lego-tray-middle-short (Autodesk Fusion 360 design; units mm, degrees)
Autodesk Fusion 360 part; units mm, degrees
sketch "Sketch1" plane through (0, 0, 0) normal (0, 1, 0) x (1, 0, 0)
  line L0 (0, 0) -> (-127, 0)
  line L1 (-127, 0) -> (-127, 103.0224)
  line L2 (-127, 103.0224) -> (0, 103.0224)
  line L3 (0, 103.0224) -> (0, 0)
  dimension "d1" = 103.0224
  dimension "d2" = 127
  constraint horizontal L0
  constraint vertical L1
  constraint horizontal L2
  constraint vertical L3
  constraint coincident L0.start L3.end
  measures "d1" distance of L0.start L2.end
  measures "d2" distance of L0.start L0.end
extrude "Extrude1" add sketch "Sketch1" along normal blind 38.1 makes body 1
draft "Draft1" [suppressed]
fillet "Fillet1" [suppressed]
fillet "Fillet2" radius 6.35 4 edges at (-127, 19.05, -103.0224) (-127, 19.05, 0) (0, 19.05, 0) (0, 19.05, -103.0224) on bodies 1
fillet "Fillet3" radius 3.175 8 edges at (-125.1401, 0, -1.8599) (-127, 0, -51.5112) (-125.1401, 0, -101.1625) (-63.5, 0, -103.0224) (-1.8599, 0, -101.1625) (0, 0, -51.5112) (-1.8599, 0, -1.8599) (-63.5, 0, 0) on bodies 1
shell "Shell1" thickness 1.524 removed faces 1 at (-44.45, 38.1, -34.3408) on bodies 1
sketch "Sketch2" plane through (0, 38.1, 0) normal (0, 1, 0) x (-1, 0, 0)
  arc A0 (6.35, -1.524) -> (1.524, -6.35) centre (6.35, -6.35) ccw
  line L0 (6.35, -1.524) -> (120.65, -1.524)
  arc A1 (125.476, -6.35) -> (120.65, -1.524) centre (120.65, -6.35) ccw
  line L1 (125.476, -6.35) -> (125.476, -96.6724)
  arc A2 (120.65, -101.4984) -> (125.476, -96.6724) centre (120.65, -96.6724) ccw
  line L2 (120.65, -101.4984) -> (6.35, -101.4984)
  arc A3 (1.524, -96.6724) -> (6.35, -101.4984) centre (6.35, -96.6724) ccw
  line L3 (1.524, -96.6724) -> (1.524, -6.35)
  arc A4 (0, -96.6724) -> (6.35, -103.0224) centre (6.35, -96.6724) ccw
  line L4 (6.35, -103.0224) -> (120.65, -103.0224)
  arc A5 (120.65, -103.0224) -> (127, -96.6724) centre (120.65, -96.6724) ccw
  line L5 (127, -96.6724) -> (127, -6.35)
  arc A6 (127, -6.35) -> (120.65, 0) centre (120.65, -6.35) ccw
  line L6 (120.65, 0) -> (6.35, 0)
  arc A7 (6.35, 0) -> (0, -6.35) centre (6.35, -6.35) ccw
  line L7 (0, -6.35) -> (0, -96.6724)
  line L8 (69.85, -1.524) -> (107.95, -1.524)
  line L9 (107.95, -1.524) -> (107.95, 0)
  line L10 (107.95, 0) -> (69.85, 0)
  line L11 (69.85, 0) -> (69.85, -1.524)
  line L12 (57.15, -103.0224) -> (19.05, -103.0224)
  line L13 (19.05, -103.0224) -> (19.05, -101.4984)
  line L14 (19.05, -101.4984) -> (57.15, -101.4984)
  line L15 (57.15, -101.4984) -> (57.15, -103.0224)
  line L16 (127, -52.2224) -> (125.476, -52.2224)
  line L17 (125.476, -52.2224) -> (125.476, -83.9724)
  line L18 (125.476, -83.9724) -> (127, -83.9724)
  line L19 (127, -83.9724) -> (127, -52.2224)
  line L20 (1.524, -50.8) -> (0, -50.8)
  line L21 (0, -50.8) -> (0, -19.05)
  line L22 (0, -19.05) -> (1.524, -19.05)
  line L23 (1.524, -19.05) -> (1.524, -50.8)
  dimension "d15" = 38.1
  dimension "d18" = 31.75
  dimension "d26" = 12.7
  dimension "d27" = 12.7
  dimension "d28" = 12.7
  dimension "d29" = 12.7
  constraint horizontal L8
  constraint vertical L9
  constraint horizontal L10
  constraint vertical L11
  constraint coincident L6 L9.end
  constraint coincident L0 L8.start
  constraint horizontal L12
  constraint vertical L13
  constraint horizontal L14
  constraint vertical L15
  constraint coincident L2 L13.end
  constraint coincident L4 L12.start
  constraint equal L8 L14
  constraint horizontal L16
  constraint vertical L17
  constraint horizontal L18
  constraint vertical L19
  constraint coincident L1 L17.end
  constraint coincident L5 L16.start
  constraint horizontal L20
  constraint vertical L21
  constraint horizontal L22
  constraint vertical L23
  constraint coincident L7 L21.end
  constraint coincident L3 L20.start
  constraint equal L19 L21
  measures "d15" distance of L9.end L10.end
  measures "d18" distance of L16.start L18.end
  measures "d26" distance of A4.end L12.end
  measures "d27" distance of A7.end L21.end
  measures "d28" distance of A6.end L9.end
  measures "d29" distance of A5.end L18.end
extrude "Extrude2" cut sketch "Sketch2" against normal blind 12.7 contours L0 L6 L8 L9 L10 L11 | L3 L7 L20 L21 L22 L23 | L1 L5 L16 L17 L18 L19 | L2 L4 L12 L13 L14 L15 bodies 1
draft "Draft2" angle 30 neutral plane through (0, 25.4, 0) pull (0, 1, 0) 8 faces at (-107.95, 33.8667, -1.016) (-69.85, 33.8667, -0.508) (-1.016, 33.8667, -50.8) (-0.508, 33.8667, -19.05) (-19.05, 33.8667, -102.5144) (-57.15, 33.8667, -102.0064) (-126.492, 33.8667, -52.2224) (-125.984, 33.8667, -83.9724) on bodies 1
fillet "Fillet4" radius 6.35 16 edges at (-126.238, 38.1, -44.8901) (-126.238, 25.4, -83.9724) (-126.238, 38.1, -91.3047) (-126.238, 25.4, -52.2224) (-64.4823, 38.1, -102.2604) (-57.15, 25.4, -102.2604) (-19.05, 25.4, -102.2604) (-11.7177, 38.1, -102.2604) (-0.762, 38.1, -58.1323) (-0.762, 25.4, -50.8) (-0.762, 38.1, -11.7177) (-0.762, 25.4, -19.05) (-62.5177, 38.1, -0.762) (-69.85, 25.4, -0.762) (-107.95, 25.4, -0.762) (-115.2823, 38.1, -0.762) on bodies 1
sketch "Sketch3" plane through (0, 1.524, 0) normal (0, 1, 0) x (-1, 0, 0)
  line L0 (123.9448, -4.0087) -> (4.0087, -100.2026)
  line L1 (4.0087, -100.2026) -> (3.0552, -99.0137)
  line L2 (3.0552, -99.0137) -> (122.9913, -2.8198)
  line L3 (122.9913, -2.8198) -> (123.9448, -4.0087)
  line L4 (123.9448, -99.0137) -> (122.9913, -100.2026)
  line L5 (122.9913, -100.2026) -> (3.0552, -4.0087)
  line L6 (3.0552, -4.0087) -> (4.0087, -2.8198)
  line L7 (4.0087, -2.8198) -> (123.9448, -99.0137)
  line L8 (63.9768, -50.9168) -> (63.9768, -52.1056) construction
  line L9 (63.9768, -52.1056) -> (63.0232, -52.1056) construction
  line L10 (63.0232, -52.1056) -> (63.0232, -50.9168) construction
  line L11 (63.0232, -50.9168) -> (63.9768, -50.9168) construction
  line L12 (6.35, -1.524) -> (58.8515, -1.524)
  line L13 (1.524, -22.7162) -> (1.524, -47.1338)
  line L14 (22.7162, -101.4984) -> (53.4838, -101.4984)
  line L15 (125.476, -6.35) -> (125.476, -41.2239)
  arc A0 (125.476, -6.35) -> (120.65, -1.524) centre (120.65, -6.35) ccw
  line L16 (123.4681, -3.4143) -> (124.0625, -2.9375) construction
  arc A1 (1.524, -96.6724) -> (6.35, -101.4984) centre (6.35, -96.6724) ccw
  line L17 (3.5319, -99.6081) -> (2.9375, -100.0849) construction
  arc A2 (6.35, -1.524) -> (1.524, -6.35) centre (6.35, -6.35) ccw
  line L18 (2.9375, -2.9375) -> (3.5319, -3.4143) construction
  point P0 (63.9768, -52.1056)
  point P1 (63.9768, -50.9168)
  point P2 (63.0232, -52.1056)
  point P3 (63.0232, -50.9168)
  point P4 (124.0625, -2.9375)
  dimension "d34" = 1.524
  dimension "d42" = 0.762
  constraint equal L3 L4
  constraint coincident L0 P0
  constraint coincident L7 P1
  constraint midpoint L7 P1
  constraint midpoint L0 P0
  constraint perpendicular L8 L9
  constraint parallel L8 L10
  constraint parallel L9 L11
  constraint coincident P0 L8.end
  constraint coincident P1 L8.start
  constraint coincident L5 P2
  constraint coincident L2 P3
  constraint midpoint L2 P3
  constraint midpoint L5 P2
  constraint coincident P3 L10.end
  constraint coincident P2 L9.end
  constraint perpendicular L0 L3
  constraint perpendicular L6 L7
  constraint perpendicular L0 L1
  constraint perpendicular L4 L5
  constraint parallel L0 L2
  constraint parallel L5 L7
  constraint horizontal L2.end L6.end
  constraint midpoint A0 P4
  constraint midpoint L3 L16.start
  constraint coincident P4 L16.end
  constraint perpendicular L3 L16
  constraint midpoint L1 L17.start
  constraint midpoint A1 L17.end
  constraint perpendicular L1 L17
  constraint equal L16 L17
  constraint midpoint A2 L18.start
  constraint midpoint L6 L18.end
  constraint perpendicular L6 L18
  measures "d34" distance of L0.start L2.end
  measures "d42" distance of L3 P4
extrude "Extrude4" add sketch "Sketch3" along normal blind 19.05 separate body contours L0 L4 L5 L7 | L0 L2 L5 L7 | L2 L5 L6 L7 makes body 2
fillet "Fillet8" radius 1.5875 4 edges at (-3.5319, 1.524, -3.4143) (-123.4681, 20.574, -99.6081) (-3.5319, 20.574, -3.4143) (-123.4681, 1.524, -99.6081) on bodies 2
sketch "Sketch4" plane through (0, 20.574, 0) normal (0, 1, 0) x (-1, 0, 0)
  line L0 (63.805, -52.7326) -> (62.2415, -51.4786)
  line L1 (62.2415, -51.4786) -> (63.195, -50.2898)
  line L2 (63.195, -50.2898) -> (64.7585, -51.5438)
  line L3 (64.7585, -51.5438) -> (63.805, -52.7326)
  line L4 (122.9913, -100.2026) -> (3.0552, -4.0087)
  line L5 (4.0087, -2.8198) -> (123.9448, -99.0137)
  line L6 (3.0552, -99.0137) -> (122.9913, -2.8198)
  line L7 (123.9448, -4.0087) -> (4.0087, -100.2026)
  dimension "d49" = 0.0508
  dimension "d50" = 0.0508
  constraint perpendicular L0 L1
  constraint parallel L0 L2
  constraint parallel L1 L3
  constraint collinear L0 L4
  constraint collinear L2 L5
  measures "d49" distance of L0.end L6
  measures "d50" distance of L2.end L7
extrude "Extrude5" cut sketch "Sketch4" against normal blind 9.525 bodies 2
copy_body "CopyPasteBodies1" bodies 2 makes body 3
move_body "Move1" bodies 3 to x (0.217084, 0, 0.976153) y (0, -1, 0) z (0.976153, 0, -0.217084) at (-0.3859, 3.048, 0.4811)
move_body "Move2" bodies 3 to x (1, 0, 0) y (0, 1, 0) z (0, 0, 1) at (0.9535, 19.05, -1.1889)
move_body "Move3" bodies 3 to x (0.21644, 0, -0.976296) y (0, 1, 0) z (0.976296, 0, 0.21644) at (-0.4194, 0, -101.1021)
move_body "Move4" bodies 3 to x (1, 0, 0) y (0, 1, 0) z (0, 0, 1) at (0.9535, 0, -1.3208)
copy_body "Body->Comp1" bodies 3 removing the originals makes body 4 in component "Component"
copy_body "Body->Comp2" bodies 2 removing the originals makes body 5 in component "Component'"
component "Component" placed x (1, 0, 0) y (0, 1, 0) z (0, 0, 1) at (0, 0, 0)
component "Component'" placed x (1, 0, 0) y (0, 1, 0) z (0, 0, 1) at (0, 0, 0)
equation "d1 = 4.071 in - 0.015 in"
equation "d2 = 5.015 in - 0.015 in"
